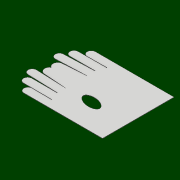
# Autodesk Inventor part: Part1
Saved by Autodesk Inventor 2018 (Build 220112000, 112)
## iProperties
Created: 2021-12-12
Part Number: Part1
Material: 一般
Document SubType Name: Modeling
Designer: gisen
Density: 1 g/cm^3
Appearance: 既定
Author: gisen
Autodesk Inventor part; units mm, degrees
ref_plane "YZ Plane" through (0, 0, 0) normal (1, 0, 0) x (0, 1, 0)
ref_plane "XZ Plane" through (0, 0, 0) normal (0, 1, 0) x (-1, 0, 0)
ref_plane "XY Plane" through (0, 0, 0) normal (0, 0, 1) x (1, 0, 0)
sketch "スケッチ1" plane through (0, 0, 0) normal (0, 0, 1) x (1, 0, 0)
  line L0 (204.1011, 235.7393) -> (-46.8337, 235.74)
  line L1 (-46.8337, 235.74) -> (-48.8539, 235.5765)
  line L2 (-48.8539, 235.5765) -> (-50.8529, 235.083)
  line L3 (-50.8529, 235.083) -> (-52.7172, 234.2937)
  line L4 (-52.7172, 234.2937) -> (-54.4186, 233.2366)
  line L5 (-54.4186, 233.2366) -> (-55.9307, 231.9388)
  line L6 (-55.9307, 231.9388) -> (-57.2283, 230.4266)
  line L7 (-57.2283, 230.4266) -> (-58.2853, 228.7251)
  line L8 (-58.2853, 228.7251) -> (-59.0745, 226.8607)
  line L9 (-59.0745, 226.8607) -> (-59.5679, 224.8617)
  line L10 (-59.5679, 224.8617) -> (-59.738, 222.7608)
  line L11 (-59.738, 222.7608) -> (-59.5679, 220.6601)
  line L12 (-59.5679, 220.6601) -> (-59.0745, 218.6613)
  line L13 (-59.0745, 218.6613) -> (-58.2853, 216.797)
  line L14 (-58.2853, 216.797) -> (-57.2283, 215.0958)
  line L15 (-57.2283, 215.0958) -> (-55.9306, 213.5836)
  line L16 (-55.9306, 213.5836) -> (-54.4185, 212.2861)
  line L17 (-54.4185, 212.2861) -> (-52.7171, 211.2291)
  line L18 (-52.7171, 211.2291) -> (-50.8528, 210.44)
  line L19 (-50.8528, 210.44) -> (-48.8538, 209.9465)
  line L20 (-48.8538, 209.9465) -> (-46.8268, 209.7825)
  line L21 (-46.8268, 209.7825) -> (15.2101, 210.2146)
  line L22 (15.2101, 210.2146) -> (15.3598, 210.2025)
  line L23 (15.3598, 210.2025) -> (15.4278, 210.1857)
  line L24 (15.4278, 210.1857) -> (15.4928, 210.1582)
  line L25 (15.4928, 210.1582) -> (15.5546, 210.1198)
  line L26 (15.5546, 210.1198) -> (15.611, 210.0715)
  line L27 (15.611, 210.0715) -> (15.6592, 210.0155)
  line L28 (15.6592, 210.0155) -> (15.6973, 209.9545)
  line L29 (15.6973, 209.9545) -> (15.7245, 209.8906)
  line L30 (15.7245, 209.8906) -> (15.7411, 209.8235)
  line L31 (15.7411, 209.8235) -> (15.7473, 209.7477)
  line L32 (15.7473, 209.7477) -> (15.7411, 209.6708)
  line L33 (15.7411, 209.6708) -> (15.7242, 209.6025)
  line L34 (15.7242, 209.6025) -> (15.697, 209.5382)
  line L35 (15.697, 209.5382) -> (15.6594, 209.4777)
  line L36 (15.6594, 209.4777) -> (15.6121, 209.4226)
  line L37 (15.6121, 209.4226) -> (15.557, 209.3753)
  line L38 (15.557, 209.3753) -> (15.4965, 209.3377)
  line L39 (15.4965, 209.3377) -> (15.4324, 209.3106)
  line L40 (15.4324, 209.3106) -> (15.3642, 209.2938)
  line L41 (15.3642, 209.2938) -> (15.1992, 209.2804)
  line L42 (15.1992, 209.2804) -> (-74.895, 208.6521)
  line L43 (-74.895, 208.6521) -> (-76.9072, 208.4891)
  line L44 (-76.9072, 208.4891) -> (-78.9056, 207.9956)
  line L45 (-78.9056, 207.9956) -> (-80.7698, 207.2064)
  line L46 (-80.7698, 207.2064) -> (-82.4714, 206.1495)
  line L47 (-82.4714, 206.1495) -> (-83.9841, 204.8521)
  line L48 (-83.9841, 204.8521) -> (-85.2825, 203.3401)
  line L49 (-85.2825, 203.3401) -> (-86.3405, 201.6388)
  line L50 (-86.3405, 201.6388) -> (-87.1306, 199.7745)
  line L51 (-87.1306, 199.7745) -> (-87.6248, 197.7753)
  line L52 (-87.6248, 197.7753) -> (-87.7951, 195.6743)
  line L53 (-87.7951, 195.6743) -> (-87.625, 193.5733)
  line L54 (-87.625, 193.5733) -> (-87.1316, 191.5743)
  line L55 (-87.1316, 191.5743) -> (-86.3424, 189.7099)
  line L56 (-86.3424, 189.7099) -> (-85.2854, 188.0085)
  line L57 (-85.2854, 188.0085) -> (-83.9879, 186.4961)
  line L58 (-83.9879, 186.4961) -> (-82.4757, 185.1984)
  line L59 (-82.4757, 185.1984) -> (-80.7743, 184.1413)
  line L60 (-80.7743, 184.1413) -> (-78.91, 183.352)
  line L61 (-78.91, 183.352) -> (-76.911, 182.8585)
  line L62 (-76.911, 182.8585) -> (-74.8913, 182.695)
  line L63 (-74.8913, 182.695) -> (5.2803, 182.6583)
  line L64 (5.2803, 182.6583) -> (5.4392, 182.6455)
  line L65 (5.4392, 182.6455) -> (5.5077, 182.6286)
  line L66 (5.5077, 182.6286) -> (5.5719, 182.6014)
  line L67 (5.5719, 182.6014) -> (5.6323, 182.5639)
  line L68 (5.6323, 182.5639) -> (5.6873, 182.5167)
  line L69 (5.6873, 182.5167) -> (5.7345, 182.4616)
  line L70 (5.7345, 182.4616) -> (5.7722, 182.401)
  line L71 (5.7722, 182.401) -> (5.7994, 182.3366)
  line L72 (5.7994, 182.3366) -> (5.8163, 182.2679)
  line L73 (5.8163, 182.2679) -> (5.8226, 182.1901)
  line L74 (5.8226, 182.1901) -> (5.8164, 182.113)
  line L75 (5.8164, 182.113) -> (5.7996, 182.0448)
  line L76 (5.7996, 182.0448) -> (5.7724, 181.9806)
  line L77 (5.7724, 181.9806) -> (5.7347, 181.92)
  line L78 (5.7347, 181.92) -> (5.6874, 181.8648)
  line L79 (5.6874, 181.8648) -> (5.6322, 181.8174)
  line L80 (5.6322, 181.8174) -> (5.5716, 181.7798)
  line L81 (5.5716, 181.7798) -> (5.5074, 181.7526)
  line L82 (5.5074, 181.7526) -> (5.4392, 181.7358)
  line L83 (5.4392, 181.7358) -> (5.2427, 181.7199)
  line L84 (5.2427, 181.7199) -> (-90.8895, 177.9794)
  line L85 (-90.8895, 177.9794) -> (-90.8977, 177.9792)
  line L86 (-90.8977, 177.9792) -> (-90.9177, 177.9785)
  line L87 (-90.9177, 177.9785) -> (-90.9351, 177.9777)
  line L88 (-90.9351, 177.9777) -> (-90.9459, 177.9771)
  line L89 (-90.9459, 177.9771) -> (-90.957, 177.9766)
  line L90 (-90.957, 177.9766) -> (-90.9597, 177.9764)
  line L91 (-90.9597, 177.9764) -> (-91.8874, 177.9378)
  line L92 (-91.8874, 177.9378) -> (-92.5543, 177.8577)
  line L93 (-92.5543, 177.8577) -> (-97.3918, 176.2859)
  line L94 (-97.3918, 176.2859) -> (-100.1871, 173.981)
  line L95 (-100.1871, 173.981) -> (-100.703, 173.4237)
  line L96 (-100.703, 173.4237) -> (-101.3371, 172.6206)
  line L97 (-101.3371, 172.6206) -> (-101.9031, 171.775)
  line L98 (-101.9031, 171.775) -> (-102.3989, 170.8907)
  line L99 (-102.3989, 170.8907) -> (-102.8228, 169.9719)
  line L100 (-102.8228, 169.9719) -> (-103.1729, 169.0224)
  line L101 (-103.1729, 169.0224) -> (-103.4477, 168.0465)
  line L102 (-103.4477, 168.0465) -> (-103.6457, 167.0484)
  line L103 (-103.6457, 167.0484) -> (-103.7653, 166.0321)
  line L104 (-103.7653, 166.0321) -> (-103.8071, 164.9601)
  line L105 (-103.8071, 164.9601) -> (-103.6407, 162.9037)
  line L106 (-103.6407, 162.9037) -> (-103.1479, 160.9069)
  line L107 (-103.1479, 160.9069) -> (-102.3598, 159.0442)
  line L108 (-102.3598, 159.0442) -> (-101.3044, 157.3441)
  line L109 (-101.3044, 157.3441) -> (-100.0088, 155.8324)
  line L110 (-100.0088, 155.8324) -> (-98.499, 154.5347)
  line L111 (-98.499, 154.5347) -> (-96.8002, 153.4769)
  line L112 (-96.8002, 153.4769) -> (-94.9386, 152.6861)
  line L113 (-94.9386, 152.6861) -> (-92.9424, 152.1905)
  line L114 (-92.9424, 152.1905) -> (-90.9235, 152.0241)
  line L115 (-90.9235, 152.0241) -> (-90.764, 152.0241)
  line L116 (-90.764, 152.0241) -> (5.7273, 155.7788)
  line L117 (5.7273, 155.7788) -> (5.7711, 155.7752)
  line L118 (5.7711, 155.7752) -> (5.7734, 155.7733)
  line L119 (5.7734, 155.7733) -> (5.7752, 155.7711)
  line L120 (5.7752, 155.7711) -> (5.7754, 155.7697)
  line L121 (5.7754, 155.7697) -> (5.7752, 155.7679)
  line L122 (5.7752, 155.7679) -> (5.7736, 155.766)
  line L123 (5.7736, 155.766) -> (5.7715, 155.7642)
  line L124 (5.7715, 155.7642) -> (5.4008, 155.7342)
  line L125 (5.4008, 155.7342) -> (3.6079, 155.601)
  line L126 (3.6079, 155.601) -> (-1.8274, 155.1969)
  line L127 (-1.8274, 155.1969) -> (-9.8297, 154.602)
  line L128 (-9.8297, 154.602) -> (-19.5444, 153.8798)
  line L129 (-19.5444, 153.8798) -> (-30.1167, 153.0939)
  line L130 (-30.1167, 153.0939) -> (-40.6916, 152.3077)
  line L131 (-40.6916, 152.3077) -> (-50.4144, 151.585)
  line L132 (-50.4144, 151.585) -> (-58.4304, 150.989)
  line L133 (-58.4304, 150.989) -> (-63.8845, 150.5836)
  line L134 (-63.8845, 150.5836) -> (-65.8482, 150.4376)
  line L135 (-65.8482, 150.4376) -> (-65.8685, 150.4376)
  line L136 (-65.8685, 150.4376) -> (-68.2875, 150.2418)
  line L137 (-68.2875, 150.2418) -> (-70.665, 149.655)
  line L138 (-70.665, 149.655) -> (-72.8824, 148.7163)
  line L139 (-72.8824, 148.7163) -> (-74.9064, 147.4588)
  line L140 (-74.9064, 147.4588) -> (-76.7056, 145.9149)
  line L141 (-76.7056, 145.9149) -> (-78.2495, 144.1157)
  line L142 (-78.2495, 144.1157) -> (-79.5069, 142.0918)
  line L143 (-79.5069, 142.0918) -> (-80.4456, 139.8743)
  line L144 (-80.4456, 139.8743) -> (-81.0325, 137.4968)
  line L145 (-81.0325, 137.4968) -> (-81.2336, 135.0115)
  line L146 (-81.2336, 135.0115) -> (-81.0985, 132.9797)
  line L147 (-81.0985, 132.9797) -> (-80.7064, 131.0254)
  line L148 (-80.7064, 131.0254) -> (-80.0727, 129.1575)
  line L149 (-80.0727, 129.1575) -> (-79.2134, 127.3964)
  line L150 (-79.2134, 127.3964) -> (-78.144, 125.7618)
  line L151 (-78.144, 125.7618) -> (-76.8794, 124.2732)
  line L152 (-76.8794, 124.2732) -> (-75.4341, 122.9502)
  line L153 (-75.4341, 122.9502) -> (-73.8224, 121.8135)
  line L154 (-73.8224, 121.8135) -> (-73.6807, 121.7389)
  line L155 (-73.6807, 121.7389) -> (-73.8222, 121.6643)
  line L156 (-73.8222, 121.6643) -> (-75.434, 120.5277)
  line L157 (-75.434, 120.5277) -> (-76.8794, 119.2049)
  line L158 (-76.8794, 119.2049) -> (-78.144, 117.7163)
  line L159 (-78.144, 117.7163) -> (-79.2134, 116.0817)
  line L160 (-79.2134, 116.0817) -> (-80.0727, 114.3207)
  line L161 (-80.0727, 114.3207) -> (-80.7064, 112.4527)
  line L162 (-80.7064, 112.4527) -> (-81.0985, 110.4984)
  line L163 (-81.0985, 110.4984) -> (-81.2309, 108.5083)
  line L164 (-81.2309, 108.5083) -> (-81.182, 107.2559)
  line L165 (-81.182, 107.2559) -> (-81.0394, 106.0476)
  line L166 (-81.0394, 106.0476) -> (-80.8037, 104.861)
  line L167 (-80.8037, 104.861) -> (-80.4766, 103.7009)
  line L168 (-80.4766, 103.7009) -> (-80.0598, 102.5723)
  line L169 (-80.0598, 102.5723) -> (-79.5554, 101.4798)
  line L170 (-79.5554, 101.4798) -> (-78.9653, 100.4283)
  line L171 (-78.9653, 100.4283) -> (-78.2918, 99.4223)
  line L172 (-78.2918, 99.4223) -> (-77.537, 98.4664)
  line L173 (-77.537, 98.4664) -> (-76.7033, 97.5653)
  line L174 (-76.7033, 97.5653) -> (-75.8019, 96.7316)
  line L175 (-75.8019, 96.7316) -> (-74.8461, 95.9769)
  line L176 (-74.8461, 95.9769) -> (-73.8401, 95.3034)
  line L177 (-73.8401, 95.3034) -> (-72.7886, 94.7133)
  line L178 (-72.7886, 94.7133) -> (-71.6961, 94.2089)
  line L179 (-71.6961, 94.2089) -> (-70.5676, 93.7921)
  line L180 (-70.5676, 93.7921) -> (-69.4076, 93.465)
  line L181 (-69.4076, 93.465) -> (-68.2211, 93.2293)
  line L182 (-68.2211, 93.2293) -> (-67.0128, 93.0867)
  line L183 (-67.0128, 93.0867) -> (-65.8719, 93.0422)
  line L184 (-65.8719, 93.0422) -> (-63.8845, 92.8944)
  line L185 (-63.8845, 92.8944) -> (-58.4304, 92.4889)
  line L186 (-58.4304, 92.4889) -> (-50.4144, 91.8929)
  line L187 (-50.4144, 91.8929) -> (-40.6916, 91.1701)
  line L188 (-40.6916, 91.1701) -> (-30.1167, 90.3838)
  line L189 (-30.1167, 90.3838) -> (-19.5445, 89.5978)
  line L190 (-19.5445, 89.5978) -> (-9.8298, 88.8755)
  line L191 (-9.8298, 88.8755) -> (-1.8274, 88.2805)
  line L192 (-1.8274, 88.2805) -> (3.6078, 87.8764)
  line L193 (3.6078, 87.8764) -> (5.3996, 87.7432)
  line L194 (5.3996, 87.7432) -> (5.7716, 87.7131)
  line L195 (5.7716, 87.7131) -> (5.7717, 87.7131)
  line L196 (5.7717, 87.7131) -> (5.7738, 87.7112)
  line L197 (5.7738, 87.7112) -> (5.7752, 87.7095)
  line L198 (5.7752, 87.7095) -> (5.7754, 87.7083)
  line L199 (5.7754, 87.7083) -> (5.7752, 87.7066)
  line L200 (5.7752, 87.7066) -> (5.7735, 87.7047)
  line L201 (5.7735, 87.7047) -> (5.7714, 87.7028)
  line L202 (5.7714, 87.7028) -> (5.7274, 87.6992)
  line L203 (5.7274, 87.6992) -> (-90.7619, 91.4532)
  line L204 (-90.7619, 91.4532) -> (-90.9235, 91.4532)
  line L205 (-90.9235, 91.4532) -> (-92.9424, 91.2869)
  line L206 (-92.9424, 91.2869) -> (-94.9386, 90.7913)
  line L207 (-94.9386, 90.7913) -> (-96.8001, 90.0007)
  line L208 (-96.8001, 90.0007) -> (-98.4989, 88.943)
  line L209 (-98.4989, 88.943) -> (-100.0088, 87.6453)
  line L210 (-100.0088, 87.6453) -> (-101.3044, 86.1338)
  line L211 (-101.3044, 86.1338) -> (-102.3598, 84.4337)
  line L212 (-102.3598, 84.4337) -> (-103.1479, 82.5711)
  line L213 (-103.1479, 82.5711) -> (-103.6407, 80.5744)
  line L214 (-103.6407, 80.5744) -> (-103.8071, 78.518)
  line L215 (-103.8071, 78.518) -> (-103.7653, 77.446)
  line L216 (-103.7653, 77.446) -> (-103.6456, 76.4297)
  line L217 (-103.6456, 76.4297) -> (-103.4477, 75.4316)
  line L218 (-103.4477, 75.4316) -> (-103.1729, 74.4557)
  line L219 (-103.1729, 74.4557) -> (-102.8228, 73.5063)
  line L220 (-102.8228, 73.5063) -> (-102.3989, 72.5875)
  line L221 (-102.3989, 72.5875) -> (-101.9032, 71.7032)
  line L222 (-101.9032, 71.7032) -> (-101.3373, 70.8575)
  line L223 (-101.3373, 70.8575) -> (-100.7033, 70.0544)
  line L224 (-100.7033, 70.0544) -> (-100.1877, 69.497)
  line L225 (-100.1877, 69.497) -> (-97.7361, 67.5796)
  line L226 (-97.7361, 67.5796) -> (-92.1007, 65.5656)
  line L227 (-92.1007, 65.5656) -> (-91.8868, 65.54)
  line L228 (-91.8868, 65.54) -> (-90.9593, 65.5016)
  line L229 (-90.9593, 65.5016) -> (-90.9573, 65.5015)
  line L230 (-90.9573, 65.5015) -> (-90.9474, 65.501)
  line L231 (-90.9474, 65.501) -> (-90.9337, 65.5003)
  line L232 (-90.9337, 65.5003) -> (-90.9207, 65.4997)
  line L233 (-90.9207, 65.4997) -> (-90.9022, 65.499)
  line L234 (-90.9022, 65.499) -> (-90.8882, 65.4986)
  line L235 (-90.8882, 65.4986) -> (5.2427, 61.7575)
  line L236 (5.2427, 61.7575) -> (5.4394, 61.7415)
  line L237 (5.4394, 61.7415) -> (5.5077, 61.7247)
  line L238 (5.5077, 61.7247) -> (5.5719, 61.6975)
  line L239 (5.5719, 61.6975) -> (5.6324, 61.6599)
  line L240 (5.6324, 61.6599) -> (5.6875, 61.6126)
  line L241 (5.6875, 61.6126) -> (5.7348, 61.5575)
  line L242 (5.7348, 61.5575) -> (5.7724, 61.4971)
  line L243 (5.7724, 61.4971) -> (5.7995, 61.4329)
  line L244 (5.7995, 61.4329) -> (5.8164, 61.3646)
  line L245 (5.8164, 61.3646) -> (5.8226, 61.2874)
  line L246 (5.8226, 61.2874) -> (5.8164, 61.2099)
  line L247 (5.8164, 61.2099) -> (5.7995, 61.1414)
  line L248 (5.7995, 61.1414) -> (5.7722, 61.077)
  line L249 (5.7722, 61.077) -> (5.7345, 61.0163)
  line L250 (5.7345, 61.0163) -> (5.6871, 60.9611)
  line L251 (5.6871, 60.9611) -> (5.632, 60.9137)
  line L252 (5.632, 60.9137) -> (5.5715, 60.8761)
  line L253 (5.5715, 60.8761) -> (5.5074, 60.849)
  line L254 (5.5074, 60.849) -> (5.4392, 60.8322)
  line L255 (5.4392, 60.8322) -> (5.281, 60.8193)
  line L256 (5.281, 60.8193) -> (-74.8913, 60.783)
  line L257 (-74.8913, 60.783) -> (-76.9108, 60.6195)
  line L258 (-76.9108, 60.6195) -> (-78.9097, 60.126)
  line L259 (-78.9097, 60.126) -> (-80.774, 59.3367)
  line L260 (-80.774, 59.3367) -> (-82.4753, 58.2796)
  line L261 (-82.4753, 58.2796) -> (-83.9876, 56.9819)
  line L262 (-83.9876, 56.9819) -> (-85.2852, 55.4696)
  line L263 (-85.2852, 55.4696) -> (-86.3422, 53.7682)
  line L264 (-86.3422, 53.7682) -> (-87.1315, 51.9038)
  line L265 (-87.1315, 51.9038) -> (-87.625, 49.9048)
  line L266 (-87.625, 49.9048) -> (-87.7951, 47.8039)
  line L267 (-87.7951, 47.8039) -> (-87.625, 45.703)
  line L268 (-87.625, 45.703) -> (-87.1316, 43.704)
  line L269 (-87.1316, 43.704) -> (-86.3424, 41.8397)
  line L270 (-86.3424, 41.8397) -> (-85.2854, 40.1383)
  line L271 (-85.2854, 40.1383) -> (-83.9878, 38.6261)
  line L272 (-83.9878, 38.6261) -> (-82.4756, 37.3285)
  line L273 (-82.4756, 37.3285) -> (-80.7742, 36.2715)
  line L274 (-80.7742, 36.2715) -> (-78.9099, 35.4823)
  line L275 (-78.9099, 35.4823) -> (-76.9109, 34.9889)
  line L276 (-76.9109, 34.9889) -> (-74.8978, 34.8259)
  line L277 (-74.8978, 34.8259) -> (15.2441, 34.1973)
  line L278 (15.2441, 34.1973) -> (15.3312, 34.194)
  line L279 (15.3312, 34.194) -> (15.3687, 34.1896)
  line L280 (15.3687, 34.1896) -> (15.4031, 34.1828)
  line L281 (15.4031, 34.1828) -> (15.435, 34.1737)
  line L282 (15.435, 34.1737) -> (15.4654, 34.1625)
  line L283 (15.4654, 34.1625) -> (15.4949, 34.1489)
  line L284 (15.4949, 34.1489) -> (15.5242, 34.1324)
  line L285 (15.5242, 34.1324) -> (15.5536, 34.1127)
  line L286 (15.5536, 34.1127) -> (15.5835, 34.0891)
  line L287 (15.5835, 34.0891) -> (15.6127, 34.062)
  line L288 (15.6127, 34.062) -> (15.6407, 34.0318)
  line L289 (15.6407, 34.0318) -> (15.6652, 34.0008)
  line L290 (15.6652, 34.0008) -> (15.686, 33.9697)
  line L291 (15.686, 33.9697) -> (15.7035, 33.9386)
  line L292 (15.7035, 33.9386) -> (15.7181, 33.907)
  line L293 (15.7181, 33.907) -> (15.73, 33.8747)
  line L294 (15.73, 33.8747) -> (15.7395, 33.8412)
  line L295 (15.7395, 33.8412) -> (15.7464, 33.8063)
  line L296 (15.7464, 33.8063) -> (15.7506, 33.7706)
  line L297 (15.7506, 33.7706) -> (15.7411, 33.6525)
  line L298 (15.7411, 33.6525) -> (15.7242, 33.5841)
  line L299 (15.7242, 33.5841) -> (15.697, 33.5198)
  line L300 (15.697, 33.5198) -> (15.6593, 33.4591)
  line L301 (15.6593, 33.4591) -> (15.6119, 33.4039)
  line L302 (15.6119, 33.4039) -> (15.5567, 33.3565)
  line L303 (15.5567, 33.3565) -> (15.4962, 33.3189)
  line L304 (15.4962, 33.3189) -> (15.4321, 33.2918)
  line L305 (15.4321, 33.2918) -> (15.364, 33.2749)
  line L306 (15.364, 33.2749) -> (15.2131, 33.2627)
  line L307 (15.2131, 33.2627) -> (-46.8289, 33.6963)
  line L308 (-46.8289, 33.6963) -> (-48.8573, 33.532)
  line L309 (-48.8573, 33.532) -> (-50.857, 33.0383)
  line L310 (-50.857, 33.0383) -> (-52.7215, 32.2489)
  line L311 (-52.7215, 32.2489) -> (-54.4227, 31.1915)
  line L312 (-54.4227, 31.1915) -> (-55.9344, 29.8936)
  line L313 (-55.9344, 29.8936) -> (-57.2312, 28.3811)
  line L314 (-57.2312, 28.3811) -> (-58.2872, 26.6797)
  line L315 (-58.2872, 26.6797) -> (-59.0755, 24.8155)
  line L316 (-59.0755, 24.8155) -> (-59.5682, 22.8168)
  line L317 (-59.5682, 22.8168) -> (-59.7379, 20.7164)
  line L318 (-59.7379, 20.7164) -> (-59.5679, 18.6156)
  line L319 (-59.5679, 18.6156) -> (-59.0745, 16.6167)
  line L320 (-59.0745, 16.6167) -> (-58.2853, 14.7523)
  line L321 (-58.2853, 14.7523) -> (-57.2283, 13.051)
  line L322 (-57.2283, 13.051) -> (-55.9307, 11.5388)
  line L323 (-55.9307, 11.5388) -> (-54.4185, 10.2412)
  line L324 (-54.4185, 10.2412) -> (-52.7171, 9.1842)
  line L325 (-52.7171, 9.1842) -> (-50.8528, 8.395)
  line L326 (-50.8528, 8.395) -> (-48.8538, 7.9015)
  line L327 (-48.8538, 7.9015) -> (-46.8337, 7.738)
  line L328 (-46.8337, 7.738) -> (204.1011, 7.738)
  line L329 (204.1011, 7.738) -> (204.1011, 235.7393)
  line L330 (57.4509, 88.8713) -> (58.8775, 86.9541)
  line L331 (58.8775, 86.9541) -> (60.5959, 85.1084)
  line L332 (60.5959, 85.1084) -> (62.607, 83.328)
  line L333 (62.607, 83.328) -> (64.8881, 81.6335)
  line L334 (64.8881, 81.6335) -> (67.415, 80.0441)
  line L335 (67.415, 80.0441) -> (70.1629, 78.5776)
  line L336 (70.1629, 78.5776) -> (73.1064, 77.2508)
  line L337 (73.1064, 77.2508) -> (76.2203, 76.0794)
  line L338 (76.2203, 76.0794) -> (79.4793, 75.0785)
  line L339 (79.4793, 75.0785) -> (82.8583, 74.2628)
  line L340 (82.8583, 74.2628) -> (86.2805, 73.6544)
  line L341 (86.2805, 73.6544) -> (89.6671, 73.2636)
  line L342 (89.6671, 73.2636) -> (92.9893, 73.0873)
  line L343 (92.9893, 73.0873) -> (96.2179, 73.1217)
  line L344 (96.2179, 73.1217) -> (99.3233, 73.3624)
  line L345 (99.3233, 73.3624) -> (102.2756, 73.8044)
  line L346 (102.2756, 73.8044) -> (105.0449, 74.4413)
  line L347 (105.0449, 74.4413) -> (107.6013, 75.2652)
  line L348 (107.6013, 75.2652) -> (109.9156, 76.2663)
  line L349 (109.9156, 76.2663) -> (111.9915, 77.4501)
  line L350 (111.9915, 77.4501) -> (112.7936, 78.0097)
  line L351 (112.7936, 78.0097) -> (113.5478, 78.61)
  line L352 (113.5478, 78.61) -> (114.2281, 79.2304)
  line L353 (114.2281, 79.2304) -> (114.8347, 79.8681)
  line L354 (114.8347, 79.8681) -> (115.368, 80.5205)
  line L355 (115.368, 80.5205) -> (115.8288, 81.1857)
  line L356 (115.8288, 81.1857) -> (116.2183, 81.8619)
  line L357 (116.2183, 81.8619) -> (116.5378, 82.5485)
  line L358 (116.5378, 82.5485) -> (116.7886, 83.2454)
  line L359 (116.7886, 83.2454) -> (116.9719, 83.9538)
  line L360 (116.9719, 83.9538) -> (117.0883, 84.6767)
  line L361 (117.0883, 84.6767) -> (117.1381, 85.4159)
  line L362 (117.1381, 85.4159) -> (117.1209, 86.1732)
  line L363 (117.1209, 86.1732) -> (117.0355, 86.9491)
  line L364 (117.0355, 86.9491) -> (116.8803, 87.7432)
  line L365 (116.8803, 87.7432) -> (116.6536, 88.5549)
  line L366 (116.6536, 88.5549) -> (116.3539, 89.3823)
  line L367 (116.3539, 89.3823) -> (115.9797, 90.2234)
  line L368 (115.9797, 90.2234) -> (115.5299, 91.0759)
  line L369 (115.5299, 91.0759) -> (115.02, 91.91)
  line L370 (115.02, 91.91) -> (113.5935, 93.827)
  line L371 (113.5935, 93.827) -> (111.8752, 95.6726)
  line L372 (111.8752, 95.6726) -> (109.8641, 97.453)
  line L373 (109.8641, 97.453) -> (107.5829, 99.1475)
  line L374 (107.5829, 99.1475) -> (105.0559, 100.7369)
  line L375 (105.0559, 100.7369) -> (102.3079, 102.2033)
  line L376 (102.3079, 102.2033) -> (99.3643, 103.5302)
  line L377 (99.3643, 103.5302) -> (96.2503, 104.7015)
  line L378 (96.2503, 104.7015) -> (92.9914, 105.7022)
  line L379 (92.9914, 105.7022) -> (89.6123, 106.5178)
  line L380 (89.6123, 106.5178) -> (86.1899, 107.1263)
  line L381 (86.1899, 107.1263) -> (82.8032, 107.5172)
  line L382 (82.8032, 107.5172) -> (79.4809, 107.6936)
  line L383 (79.4809, 107.6936) -> (76.2523, 107.6592)
  line L384 (76.2523, 107.6592) -> (73.1469, 107.4186)
  line L385 (73.1469, 107.4186) -> (70.1946, 106.9766)
  line L386 (70.1946, 106.9766) -> (67.4254, 106.3398)
  line L387 (67.4254, 106.3398) -> (64.869, 105.5159)
  line L388 (64.869, 105.5159) -> (62.5546, 104.5149)
  line L389 (62.5546, 104.5149) -> (60.4788, 103.3313)
  line L390 (60.4788, 103.3313) -> (59.6772, 102.7718)
  line L391 (59.6772, 102.7718) -> (58.9231, 102.1715)
  line L392 (58.9231, 102.1715) -> (58.2429, 101.5511)
  line L393 (58.2429, 101.5511) -> (57.6364, 100.9134)
  line L394 (57.6364, 100.9134) -> (57.1032, 100.2609)
  line L395 (57.1032, 100.2609) -> (56.6425, 99.5957)
  line L396 (56.6425, 99.5957) -> (56.253, 98.9194)
  line L397 (56.253, 98.9194) -> (55.9335, 98.2328)
  line L398 (55.9335, 98.2328) -> (55.6826, 97.5359)
  line L399 (55.6826, 97.5359) -> (55.4994, 96.8273)
  line L400 (55.4994, 96.8273) -> (55.3828, 96.1044)
  line L401 (55.3828, 96.1044) -> (55.3329, 95.3652)
  line L402 (55.3329, 95.3652) -> (55.35, 94.608)
  line L403 (55.35, 94.608) -> (55.4354, 93.8323)
  line L404 (55.4354, 93.8323) -> (55.5905, 93.0382)
  line L405 (55.5905, 93.0382) -> (55.817, 92.2267)
  line L406 (55.817, 92.2267) -> (56.1167, 91.3994)
  line L407 (56.1167, 91.3994) -> (56.4909, 90.5582)
  line L408 (56.4909, 90.5582) -> (56.9408, 89.7057)
  line L409 (56.9408, 89.7057) -> (57.4509, 88.8713)
  line L410 (204.1011, 235.7393) -> (-46.8337, 235.74)
  line L411 (-46.8337, 235.74) -> (-48.8539, 235.5765)
  line L412 (-48.8539, 235.5765) -> (-50.8529, 235.083)
  line L413 (-50.8529, 235.083) -> (-52.7172, 234.2937)
  line L414 (-52.7172, 234.2937) -> (-54.4186, 233.2366)
  line L415 (-54.4186, 233.2366) -> (-55.9307, 231.9388)
  line L416 (-55.9307, 231.9388) -> (-57.2283, 230.4266)
  line L417 (-57.2283, 230.4266) -> (-58.2853, 228.7251)
  line L418 (-58.2853, 228.7251) -> (-59.0745, 226.8607)
  line L419 (-59.0745, 226.8607) -> (-59.5679, 224.8617)
  line L420 (-59.5679, 224.8617) -> (-59.738, 222.7608)
  line L421 (-59.738, 222.7608) -> (-59.5679, 220.6601)
  line L422 (-59.5679, 220.6601) -> (-59.0745, 218.6613)
  line L423 (-59.0745, 218.6613) -> (-58.2853, 216.797)
  line L424 (-58.2853, 216.797) -> (-57.2283, 215.0958)
  line L425 (-57.2283, 215.0958) -> (-55.9306, 213.5836)
  line L426 (-55.9306, 213.5836) -> (-54.4185, 212.2861)
  line L427 (-54.4185, 212.2861) -> (-52.7171, 211.2291)
  line L428 (-52.7171, 211.2291) -> (-50.8528, 210.44)
  line L429 (-50.8528, 210.44) -> (-48.8538, 209.9465)
  line L430 (-48.8538, 209.9465) -> (-46.8268, 209.7825)
  line L431 (-46.8268, 209.7825) -> (15.2101, 210.2146)
  line L432 (15.2101, 210.2146) -> (15.3598, 210.2025)
  line L433 (15.3598, 210.2025) -> (15.4278, 210.1857)
  line L434 (15.4278, 210.1857) -> (15.4928, 210.1582)
  line L435 (15.4928, 210.1582) -> (15.5546, 210.1198)
  line L436 (15.5546, 210.1198) -> (15.611, 210.0715)
  line L437 (15.611, 210.0715) -> (15.6592, 210.0155)
  line L438 (15.6592, 210.0155) -> (15.6973, 209.9545)
  line L439 (15.6973, 209.9545) -> (15.7245, 209.8906)
  line L440 (15.7245, 209.8906) -> (15.7411, 209.8235)
  line L441 (15.7411, 209.8235) -> (15.7473, 209.7477)
  line L442 (15.7473, 209.7477) -> (15.7411, 209.6708)
  line L443 (15.7411, 209.6708) -> (15.7242, 209.6025)
  line L444 (15.7242, 209.6025) -> (15.697, 209.5382)
  line L445 (15.697, 209.5382) -> (15.6594, 209.4777)
  line L446 (15.6594, 209.4777) -> (15.6121, 209.4226)
  line L447 (15.6121, 209.4226) -> (15.557, 209.3753)
  line L448 (15.557, 209.3753) -> (15.4965, 209.3377)
  line L449 (15.4965, 209.3377) -> (15.4324, 209.3106)
  line L450 (15.4324, 209.3106) -> (15.3642, 209.2938)
  line L451 (15.3642, 209.2938) -> (15.1992, 209.2804)
  line L452 (15.1992, 209.2804) -> (-74.895, 208.6521)
  line L453 (-74.895, 208.6521) -> (-76.9072, 208.4891)
  line L454 (-76.9072, 208.4891) -> (-78.9056, 207.9956)
  line L455 (-78.9056, 207.9956) -> (-80.7698, 207.2064)
  line L456 (-80.7698, 207.2064) -> (-82.4714, 206.1495)
  line L457 (-82.4714, 206.1495) -> (-83.9841, 204.8521)
  line L458 (-83.9841, 204.8521) -> (-85.2825, 203.3401)
  line L459 (-85.2825, 203.3401) -> (-86.3405, 201.6388)
  line L460 (-86.3405, 201.6388) -> (-87.1306, 199.7745)
  line L461 (-87.1306, 199.7745) -> (-87.6248, 197.7753)
  line L462 (-87.6248, 197.7753) -> (-87.7951, 195.6743)
  line L463 (-87.7951, 195.6743) -> (-87.625, 193.5733)
  line L464 (-87.625, 193.5733) -> (-87.1316, 191.5743)
  line L465 (-87.1316, 191.5743) -> (-86.3424, 189.7099)
  line L466 (-86.3424, 189.7099) -> (-85.2854, 188.0085)
  line L467 (-85.2854, 188.0085) -> (-83.9879, 186.4961)
  line L468 (-83.9879, 186.4961) -> (-82.4757, 185.1984)
  line L469 (-82.4757, 185.1984) -> (-80.7743, 184.1413)
  line L470 (-80.7743, 184.1413) -> (-78.91, 183.352)
  line L471 (-78.91, 183.352) -> (-76.911, 182.8585)
  line L472 (-76.911, 182.8585) -> (-74.8913, 182.695)
  line L473 (-74.8913, 182.695) -> (5.2803, 182.6583)
  line L474 (5.2803, 182.6583) -> (5.4392, 182.6455)
  line L475 (5.4392, 182.6455) -> (5.5077, 182.6286)
  line L476 (5.5077, 182.6286) -> (5.5719, 182.6014)
  line L477 (5.5719, 182.6014) -> (5.6323, 182.5639)
  line L478 (5.6323, 182.5639) -> (5.6873, 182.5167)
  line L479 (5.6873, 182.5167) -> (5.7345, 182.4616)
  line L480 (5.7345, 182.4616) -> (5.7722, 182.401)
  line L481 (5.7722, 182.401) -> (5.7994, 182.3366)
  line L482 (5.7994, 182.3366) -> (5.8163, 182.2679)
  line L483 (5.8163, 182.2679) -> (5.8226, 182.1901)
  line L484 (5.8226, 182.1901) -> (5.8164, 182.113)
  line L485 (5.8164, 182.113) -> (5.7996, 182.0448)
  line L486 (5.7996, 182.0448) -> (5.7724, 181.9806)
  line L487 (5.7724, 181.9806) -> (5.7347, 181.92)
  line L488 (5.7347, 181.92) -> (5.6874, 181.8648)
  line L489 (5.6874, 181.8648) -> (5.6322, 181.8174)
  line L490 (5.6322, 181.8174) -> (5.5716, 181.7798)
  line L491 (5.5716, 181.7798) -> (5.5074, 181.7526)
  line L492 (5.5074, 181.7526) -> (5.4392, 181.7358)
  line L493 (5.4392, 181.7358) -> (5.2427, 181.7199)
  line L494 (5.2427, 181.7199) -> (-90.8895, 177.9794)
  line L495 (-90.8895, 177.9794) -> (-90.8977, 177.9792)
  line L496 (-90.8977, 177.9792) -> (-90.9177, 177.9785)
  line L497 (-90.9177, 177.9785) -> (-90.9351, 177.9777)
  line L498 (-90.9351, 177.9777) -> (-90.9459, 177.9771)
  line L499 (-90.9459, 177.9771) -> (-90.957, 177.9766)
  line L500 (-90.957, 177.9766) -> (-90.9597, 177.9764)
  line L501 (-90.9597, 177.9764) -> (-91.8874, 177.9378)
  line L502 (-91.8874, 177.9378) -> (-92.5543, 177.8577)
  line L503 (-92.5543, 177.8577) -> (-97.3918, 176.2859)
  line L504 (-97.3918, 176.2859) -> (-100.1871, 173.981)
  line L505 (-100.1871, 173.981) -> (-100.703, 173.4237)
  line L506 (-100.703, 173.4237) -> (-101.3371, 172.6206)
  line L507 (-101.3371, 172.6206) -> (-101.9031, 171.775)
  line L508 (-101.9031, 171.775) -> (-102.3989, 170.8907)
  line L509 (-102.3989, 170.8907) -> (-102.8228, 169.9719)
  line L510 (-102.8228, 169.9719) -> (-103.1729, 169.0224)
  line L511 (-103.1729, 169.0224) -> (-103.4477, 168.0465)
  line L512 (-103.4477, 168.0465) -> (-103.6457, 167.0484)
  line L513 (-103.6457, 167.0484) -> (-103.7653, 166.0321)
  line L514 (-103.7653, 166.0321) -> (-103.8071, 164.9601)
  line L515 (-103.8071, 164.9601) -> (-103.6407, 162.9037)
  line L516 (-103.6407, 162.9037) -> (-103.1479, 160.9069)
  line L517 (-103.1479, 160.9069) -> (-102.3598, 159.0442)
  line L518 (-102.3598, 159.0442) -> (-101.3044, 157.3441)
  line L519 (-101.3044, 157.3441) -> (-100.0088, 155.8324)
  line L520 (-100.0088, 155.8324) -> (-98.499, 154.5347)
  line L521 (-98.499, 154.5347) -> (-96.8002, 153.4769)
  line L522 (-96.8002, 153.4769) -> (-94.9386, 152.6861)
  line L523 (-94.9386, 152.6861) -> (-92.9424, 152.1905)
  line L524 (-92.9424, 152.1905) -> (-90.9235, 152.0241)
  line L525 (-90.9235, 152.0241) -> (-90.764, 152.0241)
  line L526 (-90.764, 152.0241) -> (5.7273, 155.7788)
  line L527 (5.7273, 155.7788) -> (5.7711, 155.7752)
  line L528 (5.7711, 155.7752) -> (5.7734, 155.7733)
  line L529 (5.7734, 155.7733) -> (5.7752, 155.7711)
  line L530 (5.7752, 155.7711) -> (5.7754, 155.7697)
  line L531 (5.7754, 155.7697) -> (5.7752, 155.7679)
  line L532 (5.7752, 155.7679) -> (5.7736, 155.766)
  line L533 (5.7736, 155.766) -> (5.7715, 155.7642)
  line L534 (5.7715, 155.7642) -> (5.4008, 155.7342)
  line L535 (5.4008, 155.7342) -> (3.6079, 155.601)
  line L536 (3.6079, 155.601) -> (-1.8274, 155.1969)
  line L537 (-1.8274, 155.1969) -> (-9.8297, 154.602)
  line L538 (-9.8297, 154.602) -> (-19.5444, 153.8798)
  line L539 (-19.5444, 153.8798) -> (-30.1167, 153.0939)
  line L540 (-30.1167, 153.0939) -> (-40.6916, 152.3077)
  line L541 (-40.6916, 152.3077) -> (-50.4144, 151.585)
  line L542 (-50.4144, 151.585) -> (-58.4304, 150.989)
  line L543 (-58.4304, 150.989) -> (-63.8845, 150.5836)
  line L544 (-63.8845, 150.5836) -> (-65.8482, 150.4376)
  line L545 (-65.8482, 150.4376) -> (-65.8685, 150.4376)
  line L546 (-65.8685, 150.4376) -> (-68.2875, 150.2418)
  line L547 (-68.2875, 150.2418) -> (-70.665, 149.655)
  line L548 (-70.665, 149.655) -> (-72.8824, 148.7163)
  line L549 (-72.8824, 148.7163) -> (-74.9064, 147.4588)
  line L550 (-74.9064, 147.4588) -> (-76.7056, 145.9149)
  line L551 (-76.7056, 145.9149) -> (-78.2495, 144.1157)
  line L552 (-78.2495, 144.1157) -> (-79.5069, 142.0918)
  line L553 (-79.5069, 142.0918) -> (-80.4456, 139.8743)
  line L554 (-80.4456, 139.8743) -> (-81.0325, 137.4968)
  line L555 (-81.0325, 137.4968) -> (-81.2336, 135.0115)
  line L556 (-81.2336, 135.0115) -> (-81.0985, 132.9797)
  line L557 (-81.0985, 132.9797) -> (-80.7064, 131.0254)
  line L558 (-80.7064, 131.0254) -> (-80.0727, 129.1575)
  line L559 (-80.0727, 129.1575) -> (-79.2134, 127.3964)
  line L560 (-79.2134, 127.3964) -> (-78.144, 125.7618)
  line L561 (-78.144, 125.7618) -> (-76.8794, 124.2732)
  line L562 (-76.8794, 124.2732) -> (-75.4341, 122.9502)
  line L563 (-75.4341, 122.9502) -> (-73.8224, 121.8135)
  line L564 (-73.8224, 121.8135) -> (-73.6807, 121.7389)
  line L565 (-73.6807, 121.7389) -> (-73.8222, 121.6643)
  line L566 (-73.8222, 121.6643) -> (-75.434, 120.5277)
  line L567 (-75.434, 120.5277) -> (-76.8794, 119.2049)
  line L568 (-76.8794, 119.2049) -> (-78.144, 117.7163)
  line L569 (-78.144, 117.7163) -> (-79.2134, 116.0817)
  line L570 (-79.2134, 116.0817) -> (-80.0727, 114.3207)
  line L571 (-80.0727, 114.3207) -> (-80.7064, 112.4527)
  line L572 (-80.7064, 112.4527) -> (-81.0985, 110.4984)
  line L573 (-81.0985, 110.4984) -> (-81.2309, 108.5083)
  line L574 (-81.2309, 108.5083) -> (-81.182, 107.2559)
  line L575 (-81.182, 107.2559) -> (-81.0394, 106.0476)
  line L576 (-81.0394, 106.0476) -> (-80.8037, 104.861)
  line L577 (-80.8037, 104.861) -> (-80.4766, 103.7009)
  line L578 (-80.4766, 103.7009) -> (-80.0598, 102.5723)
  line L579 (-80.0598, 102.5723) -> (-79.5554, 101.4798)
  line L580 (-79.5554, 101.4798) -> (-78.9653, 100.4283)
  line L581 (-78.9653, 100.4283) -> (-78.2918, 99.4223)
  line L582 (-78.2918, 99.4223) -> (-77.537, 98.4664)
  line L583 (-77.537, 98.4664) -> (-76.7033, 97.5653)
  line L584 (-76.7033, 97.5653) -> (-75.8019, 96.7316)
  line L585 (-75.8019, 96.7316) -> (-74.8461, 95.9769)
  line L586 (-74.8461, 95.9769) -> (-73.8401, 95.3034)
  line L587 (-73.8401, 95.3034) -> (-72.7886, 94.7133)
  line L588 (-72.7886, 94.7133) -> (-71.6961, 94.2089)
  line L589 (-71.6961, 94.2089) -> (-70.5676, 93.7921)
  line L590 (-70.5676, 93.7921) -> (-69.4076, 93.465)
  line L591 (-69.4076, 93.465) -> (-68.2211, 93.2293)
  line L592 (-68.2211, 93.2293) -> (-67.0128, 93.0867)
  line L593 (-67.0128, 93.0867) -> (-65.8719, 93.0422)
  line L594 (-65.8719, 93.0422) -> (-63.8845, 92.8944)
  line L595 (-63.8845, 92.8944) -> (-58.4304, 92.4889)
  line L596 (-58.4304, 92.4889) -> (-50.4144, 91.8929)
  line L597 (-50.4144, 91.8929) -> (-40.6916, 91.1701)
  line L598 (-40.6916, 91.1701) -> (-30.1167, 90.3838)
  line L599 (-30.1167, 90.3838) -> (-19.5445, 89.5978)
  line L600 (-19.5445, 89.5978) -> (-9.8298, 88.8755)
  line L601 (-9.8298, 88.8755) -> (-1.8274, 88.2805)
  line L602 (-1.8274, 88.2805) -> (3.6078, 87.8764)
  line L603 (3.6078, 87.8764) -> (5.3996, 87.7432)
  line L604 (5.3996, 87.7432) -> (5.7716, 87.7131)
  line L605 (5.7716, 87.7131) -> (5.7717, 87.7131)
  line L606 (5.7717, 87.7131) -> (5.7738, 87.7112)
  line L607 (5.7738, 87.7112) -> (5.7752, 87.7095)
  line L608 (5.7752, 87.7095) -> (5.7754, 87.7083)
  line L609 (5.7754, 87.7083) -> (5.7752, 87.7066)
  line L610 (5.7752, 87.7066) -> (5.7735, 87.7047)
  line L611 (5.7735, 87.7047) -> (5.7714, 87.7028)
  line L612 (5.7714, 87.7028) -> (5.7274, 87.6992)
  line L613 (5.7274, 87.6992) -> (-90.7619, 91.4532)
  line L614 (-90.7619, 91.4532) -> (-90.9235, 91.4532)
  line L615 (-90.9235, 91.4532) -> (-92.9424, 91.2869)
  line L616 (-92.9424, 91.2869) -> (-94.9386, 90.7913)
  line L617 (-94.9386, 90.7913) -> (-96.8001, 90.0007)
  line L618 (-96.8001, 90.0007) -> (-98.4989, 88.943)
  line L619 (-98.4989, 88.943) -> (-100.0088, 87.6453)
  line L620 (-100.0088, 87.6453) -> (-101.3044, 86.1338)
  line L621 (-101.3044, 86.1338) -> (-102.3598, 84.4337)
  line L622 (-102.3598, 84.4337) -> (-103.1479, 82.5711)
  line L623 (-103.1479, 82.5711) -> (-103.6407, 80.5744)
  line L624 (-103.6407, 80.5744) -> (-103.8071, 78.518)
  line L625 (-103.8071, 78.518) -> (-103.7653, 77.446)
  line L626 (-103.7653, 77.446) -> (-103.6456, 76.4297)
  line L627 (-103.6456, 76.4297) -> (-103.4477, 75.4316)
  line L628 (-103.4477, 75.4316) -> (-103.1729, 74.4557)
  line L629 (-103.1729, 74.4557) -> (-102.8228, 73.5063)
  line L630 (-102.8228, 73.5063) -> (-102.3989, 72.5875)
  line L631 (-102.3989, 72.5875) -> (-101.9032, 71.7032)
  line L632 (-101.9032, 71.7032) -> (-101.3373, 70.8575)
  line L633 (-101.3373, 70.8575) -> (-100.7033, 70.0544)
  line L634 (-100.7033, 70.0544) -> (-100.1877, 69.497)
  line L635 (-100.1877, 69.497) -> (-97.7361, 67.5796)
  line L636 (-97.7361, 67.5796) -> (-92.1007, 65.5656)
  line L637 (-92.1007, 65.5656) -> (-91.8868, 65.54)
  line L638 (-91.8868, 65.54) -> (-90.9593, 65.5016)
  line L639 (-90.9593, 65.5016) -> (-90.9573, 65.5015)
  line L640 (-90.9573, 65.5015) -> (-90.9474, 65.501)
  line L641 (-90.9474, 65.501) -> (-90.9337, 65.5003)
  line L642 (-90.9337, 65.5003) -> (-90.9207, 65.4997)
  line L643 (-90.9207, 65.4997) -> (-90.9022, 65.499)
  line L644 (-90.9022, 65.499) -> (-90.8882, 65.4986)
  line L645 (-90.8882, 65.4986) -> (5.2427, 61.7575)
  line L646 (5.2427, 61.7575) -> (5.4394, 61.7415)
  line L647 (5.4394, 61.7415) -> (5.5077, 61.7247)
  line L648 (5.5077, 61.7247) -> (5.5719, 61.6975)
  line L649 (5.5719, 61.6975) -> (5.6324, 61.6599)
  line L650 (5.6324, 61.6599) -> (5.6875, 61.6126)
  line L651 (5.6875, 61.6126) -> (5.7348, 61.5575)
  line L652 (5.7348, 61.5575) -> (5.7724, 61.4971)
  line L653 (5.7724, 61.4971) -> (5.7995, 61.4329)
  line L654 (5.7995, 61.4329) -> (5.8164, 61.3646)
  line L655 (5.8164, 61.3646) -> (5.8226, 61.2874)
  line L656 (5.8226, 61.2874) -> (5.8164, 61.2099)
  line L657 (5.8164, 61.2099) -> (5.7995, 61.1414)
  line L658 (5.7995, 61.1414) -> (5.7722, 61.077)
  line L659 (5.7722, 61.077) -> (5.7345, 61.0163)
  line L660 (5.7345, 61.0163) -> (5.6871, 60.9611)
  line L661 (5.6871, 60.9611) -> (5.632, 60.9137)
  line L662 (5.632, 60.9137) -> (5.5715, 60.8761)
  line L663 (5.5715, 60.8761) -> (5.5074, 60.849)
  line L664 (5.5074, 60.849) -> (5.4392, 60.8322)
  line L665 (5.4392, 60.8322) -> (5.281, 60.8193)
  line L666 (5.281, 60.8193) -> (-74.8913, 60.783)
  line L667 (-74.8913, 60.783) -> (-76.9108, 60.6195)
  line L668 (-76.9108, 60.6195) -> (-78.9097, 60.126)
  line L669 (-78.9097, 60.126) -> (-80.774, 59.3367)
  line L670 (-80.774, 59.3367) -> (-82.4753, 58.2796)
  line L671 (-82.4753, 58.2796) -> (-83.9876, 56.9819)
  line L672 (-83.9876, 56.9819) -> (-85.2852, 55.4696)
  line L673 (-85.2852, 55.4696) -> (-86.3422, 53.7682)
  line L674 (-86.3422, 53.7682) -> (-87.1315, 51.9038)
  line L675 (-87.1315, 51.9038) -> (-87.625, 49.9048)
  line L676 (-87.625, 49.9048) -> (-87.7951, 47.8039)
  line L677 (-87.7951, 47.8039) -> (-87.625, 45.703)
  line L678 (-87.625, 45.703) -> (-87.1316, 43.704)
  line L679 (-87.1316, 43.704) -> (-86.3424, 41.8397)
  line L680 (-86.3424, 41.8397) -> (-85.2854, 40.1383)
  line L681 (-85.2854, 40.1383) -> (-83.9878, 38.6261)
  line L682 (-83.9878, 38.6261) -> (-82.4756, 37.3285)
  line L683 (-82.4756, 37.3285) -> (-80.7742, 36.2715)
  line L684 (-80.7742, 36.2715) -> (-78.9099, 35.4823)
  line L685 (-78.9099, 35.4823) -> (-76.9109, 34.9889)
  line L686 (-76.9109, 34.9889) -> (-74.8978, 34.8259)
  line L687 (-74.8978, 34.8259) -> (15.2441, 34.1973)
  line L688 (15.2441, 34.1973) -> (15.3312, 34.194)
  line L689 (15.3312, 34.194) -> (15.3687, 34.1896)
  line L690 (15.3687, 34.1896) -> (15.4031, 34.1828)
  line L691 (15.4031, 34.1828) -> (15.435, 34.1737)
  line L692 (15.435, 34.1737) -> (15.4654, 34.1625)
  line L693 (15.4654, 34.1625) -> (15.4949, 34.1489)
  line L694 (15.4949, 34.1489) -> (15.5242, 34.1324)
  line L695 (15.5242, 34.1324) -> (15.5536, 34.1127)
  line L696 (15.5536, 34.1127) -> (15.5835, 34.0891)
  line L697 (15.5835, 34.0891) -> (15.6127, 34.062)
  line L698 (15.6127, 34.062) -> (15.6407, 34.0318)
  line L699 (15.6407, 34.0318) -> (15.6652, 34.0008)
  line L700 (15.6652, 34.0008) -> (15.686, 33.9697)
  line L701 (15.686, 33.9697) -> (15.7035, 33.9386)
  line L702 (15.7035, 33.9386) -> (15.7181, 33.907)
  line L703 (15.7181, 33.907) -> (15.73, 33.8747)
  line L704 (15.73, 33.8747) -> (15.7395, 33.8412)
  line L705 (15.7395, 33.8412) -> (15.7464, 33.8063)
  line L706 (15.7464, 33.8063) -> (15.7506, 33.7706)
  line L707 (15.7506, 33.7706) -> (15.7411, 33.6525)
  line L708 (15.7411, 33.6525) -> (15.7242, 33.5841)
  line L709 (15.7242, 33.5841) -> (15.697, 33.5198)
  line L710 (15.697, 33.5198) -> (15.6593, 33.4591)
  line L711 (15.6593, 33.4591) -> (15.6119, 33.4039)
  line L712 (15.6119, 33.4039) -> (15.5567, 33.3565)
  line L713 (15.5567, 33.3565) -> (15.4962, 33.3189)
  line L714 (15.4962, 33.3189) -> (15.4321, 33.2918)
  line L715 (15.4321, 33.2918) -> (15.364, 33.2749)
  line L716 (15.364, 33.2749) -> (15.2131, 33.2627)
  line L717 (15.2131, 33.2627) -> (-46.8289, 33.6963)
  line L718 (-46.8289, 33.6963) -> (-48.8573, 33.532)
  line L719 (-48.8573, 33.532) -> (-50.857, 33.0383)
  line L720 (-50.857, 33.0383) -> (-52.7215, 32.2489)
  line L721 (-52.7215, 32.2489) -> (-54.4227, 31.1915)
  line L722 (-54.4227, 31.1915) -> (-55.9344, 29.8936)
  line L723 (-55.9344, 29.8936) -> (-57.2312, 28.3811)
  line L724 (-57.2312, 28.3811) -> (-58.2872, 26.6797)
  line L725 (-58.2872, 26.6797) -> (-59.0755, 24.8155)
  line L726 (-59.0755, 24.8155) -> (-59.5682, 22.8168)
  line L727 (-59.5682, 22.8168) -> (-59.7379, 20.7164)
  line L728 (-59.7379, 20.7164) -> (-59.5679, 18.6156)
  line L729 (-59.5679, 18.6156) -> (-59.0745, 16.6167)
  line L730 (-59.0745, 16.6167) -> (-58.2853, 14.7523)
  line L731 (-58.2853, 14.7523) -> (-57.2283, 13.051)
  line L732 (-57.2283, 13.051) -> (-55.9307, 11.5388)
  line L733 (-55.9307, 11.5388) -> (-54.4185, 10.2412)
  line L734 (-54.4185, 10.2412) -> (-52.7171, 9.1842)
  line L735 (-52.7171, 9.1842) -> (-50.8528, 8.395)
  line L736 (-50.8528, 8.395) -> (-48.8538, 7.9015)
  line L737 (-48.8538, 7.9015) -> (-46.8337, 7.738)
  line L738 (-46.8337, 7.738) -> (204.1011, 7.738)
  line L739 (204.1011, 7.738) -> (204.1011, 235.7393)
  line L740 (57.4509, 88.8713) -> (58.8775, 86.9541)
  line L741 (58.8775, 86.9541) -> (60.5959, 85.1084)
  line L742 (60.5959, 85.1084) -> (62.607, 83.328)
  line L743 (62.607, 83.328) -> (64.8881, 81.6335)
  line L744 (64.8881, 81.6335) -> (67.415, 80.0441)
  line L745 (67.415, 80.0441) -> (70.1629, 78.5776)
  line L746 (70.1629, 78.5776) -> (73.1064, 77.2508)
  line L747 (73.1064, 77.2508) -> (76.2203, 76.0794)
  line L748 (76.2203, 76.0794) -> (79.4793, 75.0785)
  line L749 (79.4793, 75.0785) -> (82.8583, 74.2628)
  line L750 (82.8583, 74.2628) -> (86.2805, 73.6544)
  line L751 (86.2805, 73.6544) -> (89.6671, 73.2636)
  line L752 (89.6671, 73.2636) -> (92.9893, 73.0873)
  line L753 (92.9893, 73.0873) -> (96.2179, 73.1217)
  line L754 (96.2179, 73.1217) -> (99.3233, 73.3624)
  line L755 (99.3233, 73.3624) -> (102.2756, 73.8044)
  line L756 (102.2756, 73.8044) -> (105.0449, 74.4413)
  line L757 (105.0449, 74.4413) -> (107.6013, 75.2652)
  line L758 (107.6013, 75.2652) -> (109.9156, 76.2663)
  line L759 (109.9156, 76.2663) -> (111.9915, 77.4501)
  line L760 (111.9915, 77.4501) -> (112.7936, 78.0097)
  line L761 (112.7936, 78.0097) -> (113.5478, 78.61)
  line L762 (113.5478, 78.61) -> (114.2281, 79.2304)
  line L763 (114.2281, 79.2304) -> (114.8347, 79.8681)
  line L764 (114.8347, 79.8681) -> (115.368, 80.5205)
  line L765 (115.368, 80.5205) -> (115.8288, 81.1857)
  line L766 (115.8288, 81.1857) -> (116.2183, 81.8619)
  line L767 (116.2183, 81.8619) -> (116.5378, 82.5485)
  line L768 (116.5378, 82.5485) -> (116.7886, 83.2454)
  line L769 (116.7886, 83.2454) -> (116.9719, 83.9538)
  line L770 (116.9719, 83.9538) -> (117.0883, 84.6767)
  line L771 (117.0883, 84.6767) -> (117.1381, 85.4159)
  line L772 (117.1381, 85.4159) -> (117.1209, 86.1732)
  line L773 (117.1209, 86.1732) -> (117.0355, 86.9491)
  line L774 (117.0355, 86.9491) -> (116.8803, 87.7432)
  line L775 (116.8803, 87.7432) -> (116.6536, 88.5549)
  line L776 (116.6536, 88.5549) -> (116.3539, 89.3823)
  line L777 (116.3539, 89.3823) -> (115.9797, 90.2234)
  line L778 (115.9797, 90.2234) -> (115.5299, 91.0759)
  line L779 (115.5299, 91.0759) -> (115.02, 91.91)
  line L780 (115.02, 91.91) -> (113.5935, 93.827)
  line L781 (113.5935, 93.827) -> (111.8752, 95.6726)
  line L782 (111.8752, 95.6726) -> (109.8641, 97.453)
  line L783 (109.8641, 97.453) -> (107.5829, 99.1475)
  line L784 (107.5829, 99.1475) -> (105.0559, 100.7369)
  line L785 (105.0559, 100.7369) -> (102.3079, 102.2033)
  line L786 (102.3079, 102.2033) -> (99.3643, 103.5302)
  line L787 (99.3643, 103.5302) -> (96.2503, 104.7015)
  line L788 (96.2503, 104.7015) -> (92.9914, 105.7022)
  line L789 (92.9914, 105.7022) -> (89.6123, 106.5178)
  line L790 (89.6123, 106.5178) -> (86.1899, 107.1263)
  line L791 (86.1899, 107.1263) -> (82.8032, 107.5172)
  line L792 (82.8032, 107.5172) -> (79.4809, 107.6936)
  line L793 (79.4809, 107.6936) -> (76.2523, 107.6592)
  line L794 (76.2523, 107.6592) -> (73.1469, 107.4186)
  line L795 (73.1469, 107.4186) -> (70.1946, 106.9766)
  line L796 (70.1946, 106.9766) -> (67.4254, 106.3398)
  line L797 (67.4254, 106.3398) -> (64.869, 105.5159)
  line L798 (64.869, 105.5159) -> (62.5546, 104.5149)
  line L799 (62.5546, 104.5149) -> (60.4788, 103.3313)
  line L800 (60.4788, 103.3313) -> (59.6772, 102.7718)
  line L801 (59.6772, 102.7718) -> (58.9231, 102.1715)
  line L802 (58.9231, 102.1715) -> (58.2429, 101.5511)
  line L803 (58.2429, 101.5511) -> (57.6364, 100.9134)
  line L804 (57.6364, 100.9134) -> (57.1032, 100.2609)
  line L805 (57.1032, 100.2609) -> (56.6425, 99.5957)
  line L806 (56.6425, 99.5957) -> (56.253, 98.9194)
  line L807 (56.253, 98.9194) -> (55.9335, 98.2328)
  line L808 (55.9335, 98.2328) -> (55.6826, 97.5359)
  line L809 (55.6826, 97.5359) -> (55.4994, 96.8273)
  line L810 (55.4994, 96.8273) -> (55.3828, 96.1044)
  line L811 (55.3828, 96.1044) -> (55.3329, 95.3652)
  line L812 (55.3329, 95.3652) -> (55.35, 94.608)
  line L813 (55.35, 94.608) -> (55.4354, 93.8323)
  line L814 (55.4354, 93.8323) -> (55.5905, 93.0382)
  line L815 (55.5905, 93.0382) -> (55.817, 92.2267)
  line L816 (55.817, 92.2267) -> (56.1167, 91.3994)
  line L817 (56.1167, 91.3994) -> (56.4909, 90.5582)
  line L818 (56.4909, 90.5582) -> (56.9408, 89.7057)
  line L819 (56.9408, 89.7057) -> (57.4509, 88.8713)
  point P0 (0, 0)
  constraints: 1640 end point
extrude "押し出し1" add sketch "スケッチ1" along normal blind 1
